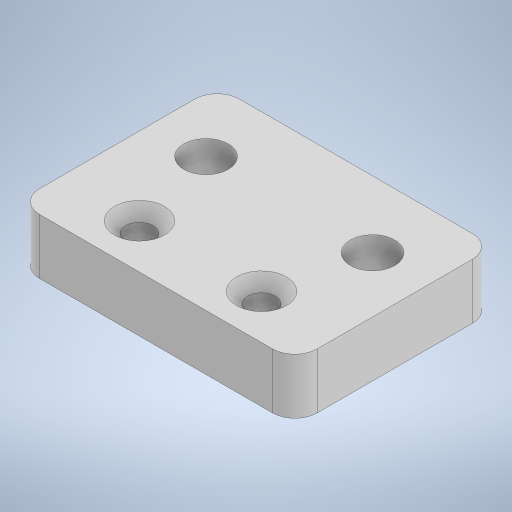
# Autodesk Inventor part: veg_kapcs_tart_csavarral
Saved by Autodesk Inventor 2024 (Build 280153000, 153)
## iProperties
Created: 2024-03-06
Part Number: veg_kapcs_tart_csavarral
Material: Generic
Document SubType Name: Modeling
Designer: Panka
Density: 1 g/cm^3
Appearance: Default
Author: Panka
Autodesk Inventor part; units mm, degrees
ref_plane "YZ Plane" through (0, 0, 0) normal (1, 0, 0) x (0, 1, 0)
ref_plane "XZ Plane" through (0, 0, 0) normal (0, 1, 0) x (-1, 0, 0)
ref_plane "XY Plane" through (0, 0, 0) normal (0, 0, 1) x (1, 0, 0)
sketch "Sketch1" plane through (0, 0, 0) normal (0, 1, 0) x (-1, 0, 0)
  line L0 (0, 0) -> (-25, 0)
  line L1 (-25, 0) -> (-25, -18)
  line L2 (-25, -18) -> (0, -18)
  line L3 (0, -18) -> (0, 0)
  circle A0 centre (-7, -4) radius 1.25
  circle A1 centre (-18, -4) radius 1.25
  circle A2 centre (-5, -12) radius 2
  circle A3 centre (-20, -12) radius 2
  dimension "d0" = 25
  dimension "d1" = 18
  dimension "d2" = 2.5
  dimension "d3" = 2.5
  dimension "d4" = 4
  dimension "d5" = 4
  dimension "d6" = 11
  dimension "d7" = 15
  dimension "d8" = 7
  dimension "d9" = 5
  dimension "d10" = 4
  dimension "d11" = 4
  dimension "d12" = 8
  constraints: 8 end point, 4 centre point, 2 parallel, 1 horizontal, 1 perpendicular
  measures "d0" distance of L2.end L1.end
  measures "d1" distance of L0.end L1.end
  measures "d2" diameter of A0
  measures "d3" diameter of A1
  measures "d4" diameter of A2
  measures "d5" diameter of A3
  measures "d6" distance of A1.centre A0.centre
  measures "d7" distance of A3.centre A2.centre
  measures "d8" distance from line of L3 A0.centre
  measures "d9" distance from line of L3 A2.centre
  measures "d10" distance from line of L0 A0.centre
  measures "d11" distance from line of L0 A1.centre
  measures "d12" vertical distance of A2.centre A0.centre
extrude "Extrusion1" add sketch "Sketch1" along normal blind 5
fillet "Fillet1" radius 2 4 edges at (0, 2.5, 0) (0, 2.5, -18) (25, 2.5, -18) (25, 2.5, 0)
chamfer "Chamfer1" distance 1 angle 45 1 edges at (8.25, 5, -4)
chamfer "Chamfer2" distance 1 angle 45 1 edges at (19.25, 5, -4)
body "Solid1"
